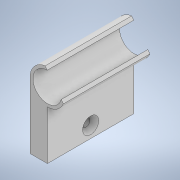
# Autodesk Inventor part: shadeHolderEmergencyExitWindow
Saved by Autodesk Inventor 2021.2 (Build 252289000, 289)
## iProperties
Created: 2021-02-12
Part Number: shadeHolderEmergencyExitWindow
Material: Generic
Document SubType Name: Modeling
Designer: robst
Density: 1 g/cm^3
Appearance: Default
Author: robst
Autodesk Inventor part; units mm, degrees
ref_plane "YZ Plane" through (0, 0, 0) normal (1, 0, 0) x (0, 1, 0)
ref_plane "XZ Plane" through (0, 0, 0) normal (0, 1, 0) x (-1, 0, 0)
ref_plane "XY Plane" through (0, 0, 0) normal (0, 0, 1) x (1, 0, 0)
sketch "Sketch4" plane through (0, 0, 0) normal (0, 0, 1) x (1, 0, 0)
  arc A0 (-0.0698, 6.3496) -> (6.1152, -1.7109) centre (0, 0) ccw
  arc A1 (-0.9946, 7.5548) -> (7.04, -2.916) centre (0, 0) ccw
  line L0 (0, 0) -> (0, 7.9375) construction
  line L1 (-0.0698, 6.3496) -> (6.1152, -1.7109) construction
  line L2 (-0.0698, 6.3496) -> (-0.9946, 7.5548)
  line L3 (6.1152, -1.7109) -> (7.04, -2.916)
  circle A2 centre (0, 0) radius 6.35
  dimension "d10" = 12.7
  dimension "d11" = 1.27
  dimension "d12" = 37.5
  dimension "d13" = 10.16
  constraints: 8 end point, 4 point on circle, 3 centre point, 3 coincident, 1 collinear, 1 concentric, 1 point on line, 1 vertical
  measures "d10" diameter of A0
  measures "d11" radial gap between concentric circles of A1 A0
  measures "d12" angle of L1 L0
  measures "d13" distance of L1.start L1.end
extrude "Extrusion3" add sketch "Sketch4" along normal mid plane 38.1 contours A0 L3 A1 L2
sketch "Sketch5" plane through (0, 0, 0) normal (0, 0, 1) x (1, 0, 0)
  arc A0 (-0.9946, 7.5548) -> (7.04, -2.916) centre (0, 0) ccw projected
  line L0 (-7.62, 0) -> (-7.62, -29.21)
  line L1 (-7.62, -29.21) -> (0, -29.21)
  line L2 (0, -29.21) -> (0, -7.62)
  circle A1 centre (0, 0) radius 7.9375
  dimension "d16" = 21.59
  constraints: 6 end point, 2 perpendicular, 2 point on circle, 1 centre point, 1 coincident, 1 tangent, 1 vertical
  measures "d16" distance from line of L2.end L1
extrude "Extrusion4" add sketch "Sketch5" along normal mid plane 38.1 contours A0 L2 A1 L0 | A1 L2 L1 L0 picked at (-7.3048, -2.4081)
sketch "Sketch6" plane through (0, -29.21, 19.05) normal (1, 0, 0) x (0, 0, -1)
  line L0 (0, 21.59) -> (38.1, 21.59) projected
  line L1 (38.1, 21.59) -> (38.1, 0) projected
  line L2 (0, 0) -> (38.1, 0) projected
  line L3 (0, 0) -> (0, 21.59) projected
  line L4 (19.05, 0) -> (19.05, 21.59) construction
  point P0 (19.05, 29.21)
  point P1 (19.05, 5.08)
  dimension "d30" = 5.08
  dimension "d31" = 0
  constraints: 2 end point, 2 midpoint
  measures "d30" distance from line of point (19.05, 5.08) L2
  measures "d31" distance from line of point (19.05, 5.08) L4
hole "Hole1" at (0, -24.13, 0) direction (-1, 0, 0) diameter 3.5052 end through all countersink diameter 7.112 countersink angle 82
sketch "Sketch10" plane through (-7.62, -29.21, 19.05) normal (0, -1, 0) x (1, 0, 0)
  line L0 (0, -38.1) -> (0, 0) projected
  line L1 (7.62, -38.1) -> (0, -38.1) projected
  line L2 (7.62, 0) -> (7.62, -38.1) projected
  line L3 (0, 0) -> (7.62, 0) projected
  line L4 (3.81, -38.1) -> (3.81, 0) construction
  spline S0 degree 2 poles (2.8014, -21.2421) (3.1307, -21.2421) (3.7235, -21.4768) (3.9294, -21.6867) knots 0 0 0 1 2 2 2
  spline S1 degree 2 poles (3.9294, -21.6867) (4.1887, -21.9502) (4.4563, -22.6624) (4.4563, -23.2058) knots 0 0 0 1 2 2 2
  line L5 (4.4563, -23.2058) -> (4.4563, -23.778)
  line L6 (4.4563, -23.778) -> (6.35, -23.778)
  line L7 (6.35, -23.778) -> (6.35, -24.4532)
  line L8 (6.35, -24.4532) -> (1.27, -24.4532)
  line L9 (1.27, -24.4532) -> (1.27, -23.177)
  spline S2 degree 2 poles (1.27, -23.177) (1.27, -22.7241) (1.4182, -22.0902) (1.587, -21.8473) knots 0 0 0 1 2 2 2
  spline S3 degree 2 poles (1.587, -21.8473) (1.7805, -21.5632) (2.3774, -21.2421) (2.8014, -21.2421) knots 0 0 0 1 2 2 2
  spline S4 degree 2 poles (2.822, -21.9461) (2.5585, -21.9461) (2.1716, -22.1272) (2.0481, -22.3125) knots 0 0 0 1 2 2 2
  spline S5 degree 2 poles (2.0481, -22.3125) (1.941, -22.473) (1.8546, -22.9012) (1.8546, -23.2182) knots 0 0 0 1 2 2 2
  line L10 (1.8546, -23.2182) -> (1.8546, -23.778)
  line L11 (1.8546, -23.778) -> (3.88, -23.778)
  line L12 (3.88, -23.778) -> (3.88, -23.317)
  spline S6 degree 2 poles (3.88, -23.317) (3.88, -22.9053) (3.7482, -22.3989) (3.5753, -22.2343) knots 0 0 0 1 2 2 2
  spline S7 degree 2 poles (3.5753, -22.2343) (3.423, -22.0819) (3.0649, -21.9461) (2.822, -21.9461) knots 0 0 0 1 2 2 2
  line L13 (1.27, -16.9155) -> (6.35, -18.6651)
  line L14 (6.35, -18.6651) -> (6.35, -19.3937)
  line L15 (6.35, -19.3937) -> (1.27, -21.1433)
  line L16 (1.27, -21.1433) -> (1.27, -20.4188)
  line L17 (1.27, -20.4188) -> (5.4896, -19.0109)
  line L18 (5.4896, -19.0109) -> (1.27, -17.603)
  line L19 (1.27, -17.603) -> (1.27, -16.9155)
  line L20 (6.35, -13.3834) -> (6.35, -16.5162)
  line L21 (6.35, -16.5162) -> (5.6296, -16.5162)
  spline S8 degree 2 poles (5.6296, -16.5162) (5.3126, -16.1786) (4.7239, -15.5776) (4.4069, -15.2894) knots 0 0 0 1 2 2 2
  spline S9 degree 2 poles (4.4069, -15.2894) (3.7688, -14.7089) (3.0031, -14.2849) (2.5956, -14.2849) knots 0 0 0 1 2 2 2
  spline S10 degree 2 poles (2.5956, -14.2849) (2.3815, -14.2849) (2.0604, -14.4167) (1.9575, -14.536) knots 0 0 0 1 2 2 2
  spline S11 degree 2 poles (1.9575, -14.536) (1.8546, -14.6554) (1.7517, -14.9683) (1.7517, -15.1577) knots 0 0 0 1 2 2 2
  spline S12 degree 2 poles (1.7517, -15.1577) (1.7517, -15.3388) (1.8422, -15.7093) (1.9122, -15.8781) knots 0 0 0 1 2 2 2
  spline S13 degree 2 poles (1.9122, -15.8781) (1.9698, -16.0222) (2.1345, -16.2898) (2.1921, -16.3721) knots 0 0 0 1 2 2 2
  line L22 (2.1921, -16.3721) -> (2.1921, -16.4091)
  line L23 (2.1921, -16.4091) -> (1.4676, -16.4091)
  spline S14 degree 2 poles (1.4676, -16.4091) (1.3647, -16.1992) (1.163, -15.4458) (1.163, -15.1083) knots 0 0 0 1 2 2 2
  spline S15 degree 2 poles (1.163, -15.1083) (1.163, -14.3961) (1.9163, -13.5933) (2.5585, -13.5933) knots 0 0 0 1 2 2 2
  spline S16 degree 2 poles (2.5585, -13.5933) (2.859, -13.5933) (3.3613, -13.7333) (3.5753, -13.8568) knots 0 0 0 1 2 2 2
  spline S17 degree 2 poles (3.5753, -13.8568) (3.7976, -13.9803) (4.234, -14.3384) (4.444, -14.536) knots 0 0 0 1 2 2 2
  spline S18 degree 2 poles (4.444, -14.536) (4.7939, -14.8571) (5.5431, -15.6434) (5.7613, -15.8781) knots 0 0 0 1 2 2 2
  line L24 (5.7613, -15.8781) -> (5.7613, -13.3834)
  line L25 (5.7613, -13.3834) -> (6.35, -13.3834)
  point P0 (7.62, -19.05)
  constraints: 2 end point, 2 midpoint, 1 vertical
extrude "Text" cut sketch "Sketch10" against normal blind 1.143 contours S0 S1 L5 L6 L7 L8 L9 S2 S3 | L13 L14 L15 L16 L17 L18 L19 | L20 L21 S8 S9 S10 S11 S12 S13 L22 L23 S14 S15 S16 S17 S18 L24 L25
equation "\"d10\" = shadeDiameter"
equation "\"d11\" = shadeHolderWallThickness"
equation "\"d13\" = openingForShade"
equation "\"d14\" = partWidth"
equation "\"d16\" = flatBelowShade"
equation "\"d17\" = partWidth"
equation "\"d30\" = holeHeightAboveBottom"
equation "\"d28\" = textDepth"
equation "\"shadeDiameter\" = 12.7"
equation "\"partWidth\" = 38.1"
equation "\"backThickness\" = 1.905"
equation "\"backHeight\" = 25.4"
equation "\"cutTiltAngle\" = 52.5deg"
equation "\"flatBelowShade\" = 21.59"
equation "\"shadeHolderWallThickness\" = 1.27"
equation "\"openingForShade\" = 10.16"
equation "\"textDepth\" = 1.143"
equation "\"holeHeightAboveBottom\" = 5.08"
body "Solid2"
